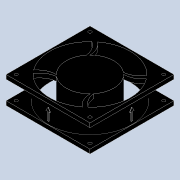
# Autodesk Inventor part: 110AC Fan
Saved by Autodesk Inventor 2022 (Build 260153000, 153)
## iProperties
Created: 2022-01-01
Part Number: 110AC Fan
Material: Generic
Document SubType Name: Modeling
Designer: Coy
Density: 1 g/cm^3
Appearance: Anodized - Black
Author: Coy
Autodesk Inventor part; units mm, degrees
ref_plane "YZ Plane" through (0, 0, 0) normal (1, 0, 0) x (0, 1, 0)
ref_plane "XZ Plane" through (0, 0, 0) normal (0, 1, 0) x (-1, 0, 0)
ref_plane "XY Plane" through (0, 0, 0) normal (0, 0, 1) x (1, 0, 0)
sketch "Sketch1" plane through (0, 0, 0) normal (0, 1, 0) x (-1, 0, 0)
  line L0 (0, 0) -> (120, 0)
  line L1 (120, 0) -> (120, 120)
  line L2 (120, 120) -> (0, 120)
  line L3 (0, 120) -> (0, 0)
  circle A0 centre (60, 60) radius 57.5
  circle A1 centre (60, 60) radius 34
  spline S0 degree 2 poles (84.1438, 36.061) (84.0562, 23.335) (94.7364, 14.1782) knots 0 0 0 1 1 1
  spline S1 degree 2 poles (86.5138, 38.7158) (87.757, 26.0504) (99.3358, 18.0602) knots 0 0 0 1 1 1
  spline S2 degree 2 poles (83.939, 84.1438) (96.665, 84.0562) (105.8218, 94.7364) knots 0 0 0 1 1 1
  spline S3 degree 2 poles (81.2842, 86.5138) (93.9496, 87.757) (101.9398, 99.3358) knots 0 0 0 1 1 1
  spline S4 degree 2 poles (35.8562, 83.939) (35.9438, 96.665) (25.2636, 105.8218) knots 0 0 0 1 1 1
  spline S5 degree 2 poles (33.4862, 81.2842) (32.243, 93.9496) (20.6642, 101.9398) knots 0 0 0 1 1 1
  spline S6 degree 2 poles (36.061, 35.8562) (23.335, 35.9438) (14.1782, 25.2636) knots 0 0 0 1 1 1
  spline S7 degree 2 poles (38.7158, 33.4862) (26.0504, 32.243) (18.0602, 20.6642) knots 0 0 0 1 1 1
  point P0 (86.6046, 24.5288)
  point P1 (90.1666, 27.504)
  point P2 (95.4712, 86.6046)
  point P3 (92.496, 90.1666)
  point P4 (33.3954, 95.4712)
  point P5 (29.8334, 92.496)
  point P6 (24.5288, 33.3954)
  point P7 (27.504, 29.8334)
  point P8 (18.0602, 20.6642)
  point P9 (38.7158, 33.4862)
  point P10 (86.5138, 38.7158)
  point P11 (105.8218, 94.7364)
  point P12 (99.3358, 18.0602)
  point P13 (25.2636, 105.8218)
  point P14 (101.9398, 99.3358)
  point P15 (36.061, 35.8562)
  point P16 (14.1782, 25.2636)
  point P17 (20.6642, 101.9398)
  dimension "d2" = 115
  dimension "d3" = 68
  dimension "d0" = 120
  dimension "d1" = 120
  dimension "d6" = 6
  dimension "d10" = 360
  constraints: 8 end point, 2 parallel, 1 coincident, 1 horizontal, 1 perpendicular, 68 other
  measures "d0" distance of L2.end L1.end
  measures "d1" distance of L1.end L0.end
extrude "Extrusion1" add sketch "Sketch1" against normal blind 6 contours L3 L2 L1 L0 | S2 A1 S3 A0 | A0 S0 A1 S1 | A1 | S4 A1 S5 A0 | A0 S6 A1 S7
sketch "Sketch2" plane through (0, -6, 0) normal (0, -1, 0) x (1, 0, 0)
  line L0 (-120, 120) -> (-120, 0) projected
  line L1 (-120, 0) -> (0, 0) projected
  line L2 (0, 0) -> (0, 120) projected
  line L3 (0, 120) -> (-120, 120) projected
  arc A0 (-84.1438, 36.061) -> (-38.7158, 33.4862) centre (-60, 60) ccw projected
  arc A1 (-94.7364, 14.1782) -> (-18.0602, 20.6642) centre (-60, 60) ccw projected
  arc A2 (-83.939, 84.1438) -> (-86.5138, 38.7158) centre (-60, 60) ccw projected
  arc A3 (-105.8218, 94.7364) -> (-99.3358, 18.0602) centre (-60, 60) ccw projected
  arc A4 (-35.8562, 83.939) -> (-81.2842, 86.5138) centre (-60, 60) ccw projected
  arc A5 (-25.2636, 105.8218) -> (-101.9398, 99.3358) centre (-60, 60) ccw projected
  arc A6 (-36.061, 35.8562) -> (-33.4862, 81.2842) centre (-60, 60) ccw projected
  arc A7 (-14.1782, 25.2636) -> (-20.6642, 101.9398) centre (-60, 60) ccw projected
  circle A8 centre (-60, 60) radius 34
  circle A9 centre (-60, 60) radius 57.5
  circle A10 centre (-60, 60) radius 59.5
  point P0 (-38.7158, 33.4862)
  point P1 (-36.061, 35.8562)
  point P2 (-33.4862, 81.2842)
  point P3 (-35.8562, 83.939)
  point P4 (-84.1438, 36.061)
  point P5 (-94.7364, 14.1782)
  point P6 (-101.9398, 99.3358)
  point P7 (-25.2636, 105.8218)
  point P8 (-20.6642, 101.9398)
  point P9 (-14.1782, 25.2636)
  point P10 (-18.0602, 20.6642)
  dimension "d14" = 2
  constraints: 2 coincident, 1 centre point, 14 other
extrude "Extrusion2" add sketch "Sketch2" along normal blind 26.5 contours A8 A2 A4 A6 A0 | A10
sketch "Sketch3" plane through (-60, -32.5, 60) normal (0, -1, 0) x (1, 0, 0)
  line L0 (-60, 60) -> (-60, -60) projected
  line L1 (-60, -60) -> (60, -60) projected
  line L2 (60, -60) -> (60, 60) projected
  line L3 (60, 60) -> (-60, 60) projected
  circle A0 centre (0, 0) radius 59.5 projected
  circle A1 centre (0, 0) radius 59.5 projected
  circle A2 centre (0, 0) radius 57.5 projected
  circle A3 centre (0, 0) radius 34 projected
extrude "Extrusion3" add sketch "Sketch3" along normal blind 6 contours L3 L2 L1 L0 | A0 | A3
sketch "Sketch4" plane through (0, 0, 0) normal (0, 1, 0) x (1, 0, 0)
  line L0 (-7.25, -112.75) -> (-112.75, -112.75) construction
  line L1 (-112.75, -112.75) -> (-112.75, -7.25) construction
  line L2 (-112.75, -7.25) -> (-7.25, -7.25) construction
  line L3 (-7.25, -7.25) -> (-7.25, -112.75) construction
  line L4 (-7.25, -112.75) -> (-7.25, -120) construction
  line L5 (-120, -120) -> (0, -120) construction
  line L6 (-7.25, -112.75) -> (0, -112.75) construction
  line L7 (0, 0) -> (0, -120) construction
  line L8 (-112.75, -7.25) -> (-112.75, 0) construction
  line L9 (-120, 0) -> (0, 0) construction
  line L10 (-112.75, -7.25) -> (-120, -7.25) construction
  line L11 (-120, -120) -> (-120, 0) construction
  circle A0 centre (-7.25, -112.75) radius 2.25
  circle A1 centre (-112.75, -112.75) radius 2.25
  circle A2 centre (-112.75, -7.25) radius 2.25
  circle A3 centre (-7.25, -7.25) radius 2.25
  dimension "d19" = 105.5
  dimension "d20" = 105.5
  dimension "d21" = 4.5
  dimension "d22" = 4.5
  dimension "d23" = 4.5
  dimension "d24" = 4.5
  constraints: 16 end point, 4 centre point, 4 coincident, 4 parallel, 4 perpendicular, 4 point on line, 1 horizontal, 1 vertical
  measures "d19" distance of L0.start L0.end
  measures "d20" distance of L0.end L1.end
  measures "d21" diameter of A0
  measures "d22" diameter of A1
  measures "d23" diameter of A2
  measures "d24" diameter of A3
extrude "Extrusion4" cut sketch "Sketch4" against normal through all
sketch "Sketch5" plane through (-120, 0, 0) normal (-1, 0, 0) x (0, 0, 1)
  line L0 (120, -38.5) -> (0, -38.5) construction
  line L1 (60, -38.5) -> (60, 0) construction
  line L2 (0, 0) -> (120, 0) construction
  line L3 (61, -15.75) -> (61, -27.75)
  line L4 (61, -27.75) -> (59, -27.75)
  line L5 (59, -27.75) -> (59, -15.75)
  line L6 (59, -15.75) -> (61, -27.75) construction
  line L7 (61, -15.75) -> (59, -27.75) construction
  line L8 (59, -15.75) -> (57, -15.75)
  line L9 (61, -15.75) -> (63, -15.75)
  line L10 (63, -15.75) -> (60, -10.75)
  line L11 (57, -15.75) -> (60, -10.75)
  line L12 (120, -32.5) -> (0, -32.5) projected
  point P0 (60, -21.75)
  dimension "d27" = 2
  dimension "d28" = 12
  dimension "d29" = 2
  dimension "d30" = 2
  dimension "d31" = 4.75
  dimension "d32" = 12
  dimension "d33" = 12
  dimension "d34" = 17
  constraints: 20 end point, 4 midpoint, 2 perpendicular, 2 point on line, 1 parallel
  measures "d27" distance of L3.end L4.end
  measures "d28" distance of L3.start L3.end
  measures "d29" distance of L5.end L8.end
  measures "d30" distance of L3.start L9.end
  measures "d31" distance between parallel lines of L12 L4
  measures "d32" distance from line of L3.end L9
  measures "d33" distance from line of L4.end L8
  measures "d34" distance from line of L4 L10.end
extrude "Extrusion5" add sketch "Sketch5" against normal up to next
pattern_circular "Circular Pattern1" count 4 over 360 about axis through (-60, 0, 60) along (0, -1, 0) of "Extrusion5"
equation "\"d0\" = d1"
equation "\"d20\" = d19"
equation "\"d22\" = d21"
equation "\"d23\" = d21"
equation "\"d24\" = d21"
body "Solid1"
